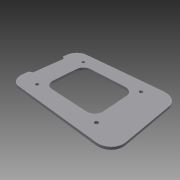
# Autodesk Inventor part: WarBRD_Upper_Plate
Saved by Autodesk Inventor 2014 SP1 (Build 180222100, 222)
## iProperties
Created: 2020-04-11
Part Number: WarBRD_Upper_Plate
Material: Všeobecné
Document SubType Name: Modeling
Designer: Jozko Mrkvicka
Density: 1 g/cm^3
Appearance: Výchozí
Author: Jozko Mrkvicka
Autodesk Inventor part; units mm, degrees
ref_plane "YZ Plane" through (0, 0, 0) normal (1, 0, 0) x (0, 1, 0)
ref_plane "XZ Plane" through (0, 0, 0) normal (0, 1, 0) x (-1, 0, 0)
ref_plane "XY Plane" through (0, 0, 0) normal (0, 0, 1) x (1, 0, 0)
sketch "Náčrt1" plane through (0, 0, 0) normal (0, 0, 1) x (1, 0, 0)
  line L0 (15, 0) -> (115, 0)
  line L1 (130, 15) -> (130, 73)
  line L2 (115, 88) -> (15, 88)
  line L3 (40.5, 69) -> (85.5, 69)
  line L4 (95.5, 59) -> (95.5, 29)
  line L5 (85.5, 19) -> (40.5, 19)
  line L6 (30.5, 29) -> (30.5, 59)
  arc A0 (40.5, 69) -> (30.5, 59) centre (40.5, 59) ccw
  arc A1 (95.5, 59) -> (85.5, 69) centre (85.5, 59) ccw
  arc A2 (85.5, 19) -> (95.5, 29) centre (85.5, 29) ccw
  arc A3 (30.5, 29) -> (40.5, 19) centre (40.5, 29) ccw
  arc A4 (130, 73) -> (115, 88) centre (115, 73) ccw
  arc A5 (115, 0) -> (130, 15) centre (115, 15) ccw
  arc A6 (15, 88) -> (0, 73) centre (15, 73) ccw
  arc A7 (0, 15) -> (15, 0) centre (15, 15) ccw
  circle A8 centre (25, 74) radius 2
  circle A9 centre (25, 14) radius 2
  circle A10 centre (101, 73) radius 2
  circle A11 centre (101, 15.1524) radius 2
  line L7 (4.5, 64) -> (4.5, 24)
  line L8 (4.5, 64) -> (0, 66.5981)
  line L9 (4.5, 24) -> (0, 21.4019)
  line L10 (0, 73) -> (0, 66.5981)
  line L11 (0, 21.4019) -> (0, 15)
  point P0 (0, 0)
  point P1 (30.5, 69)
  point P2 (95.5, 69)
  point P3 (30.5, 19)
  dimension "d0" = 65
  dimension "d1" = 50
  dimension "d7" = 34.5
  dimension "d9" = 88
  dimension "d10" = 19
  dimension "d16" = 76
  dimension "d18" = 60
  dimension "d19" = 14
  dimension "d23" = 105
  dimension "d24" = 0
  constraints: 24 end point, 18 tangent, 16 point on circle, 12 centre point, 7 point on line, 5 parallel, 3 equal radius, 2 horizontal, 2 perpendicular
  measures "d0" distance of point (30.5, 69) point (95.5, 69)
  measures "d1" distance of point (30.5, 19) point (30.5, 69)
  measures "d7" distance between parallel lines of L1 L4
  measures "d9" distance between parallel lines of L0 L2
  measures "d10" distance between parallel lines of L0 L5
  measures "d16" horizontal distance of A10.centre A8.centre
  measures "d18" distance of A8.centre A9.centre
  measures "d19" distance from line of L0 A9.centre
  measures "d23" distance from line of A8.centre L1
  measures "d24" horizontal distance of A11.centre A10.centre
extrude "Vysunutí1" add sketch "Náčrt1" along normal blind 3
